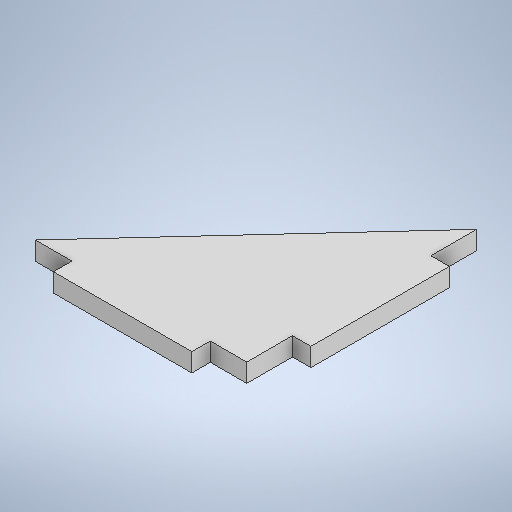
# Autodesk Inventor part: sensor_supporter
Saved by Autodesk Inventor 2025 (Build 290162000, 162)
## iProperties
Created: 2024-05-11
Part Number: sensor_supporter
Material: 일반
Document SubType Name: Modeling
Designer: gmsee
Density: 1 g/cm^3
Appearance: 기본값
Author: gmsee
Autodesk Inventor part; units mm, degrees
ref_plane "YZ Plane" through (0, 0, 0) normal (1, 0, 0) x (0, 1, 0)
ref_plane "XZ Plane" through (0, 0, 0) normal (0, 1, 0) x (-1, 0, 0)
ref_plane "XY Plane" through (0, 0, 0) normal (0, 0, 1) x (1, 0, 0)
sketch "스케치1" plane through (0, 0, 0) normal (0, 1, 0) x (-1, 0, 0)
  line L0 (23.9664, 18.1446) -> (-6.0336, 18.1446)
  line L1 (-6.0336, 18.1446) -> (-6.0336, 14.1446)
  line L2 (-6.0336, 14.1446) -> (-13.9336, 14.1446)
  line L3 (-13.9336, 14.1446) -> (-13.9336, 4.2446)
  line L4 (-13.9336, 4.2446) -> (-17.9336, 4.2446)
  line L5 (-17.9336, 4.2446) -> (-17.9336, -25.7554)
  line L6 (-17.9336, -25.7554) -> (-13.9336, -25.7554)
  line L7 (-13.9336, -25.7554) -> (-13.9336, -35.6554)
  line L8 (-13.9336, -35.6554) -> (31.8664, 14.1446)
  line L9 (31.8664, 14.1446) -> (23.9664, 14.1446)
  line L10 (23.9664, 18.1446) -> (23.9664, 14.1446)
  point P0 (0, 0)
  dimension "d0" = 7.9
  dimension "d1" = 7.9
  dimension "d2" = 30
  dimension "d3" = 4
  dimension "d4" = 4
  dimension "d5" = 9.9
  dimension "d6" = 9.9
  dimension "d7" = 30
  constraints: 22 end point, 6 perpendicular, 4 point on line, 1 horizontal, 1 vertical
  measures "d0" distance of L1.end L2.end
  measures "d1" distance of L8.end L9.end
  measures "d2" distance of L0.start L0.end
  measures "d3" distance of L0.end L1.end
  measures "d4" distance of L3.end L4.end
  measures "d5" distance of L2.end L3.end
  measures "d6" distance of L6.end L7.end
  measures "d7" distance of L4.end L5.end
extrude "돌출1" add sketch "스케치1" along normal blind 4
